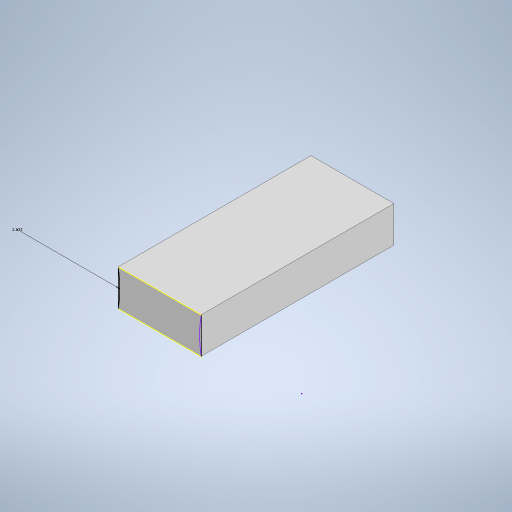
# Autodesk Inventor part: T610
Saved by Autodesk Inventor 2023 (Build 270158000, 158)
## iProperties
Created: 2023-01-25
Part Number: T610
Material: Generic
Document SubType Name: Modeling
Designer: abhim
Density: 1 g/cm^3
Appearance: Default
Author: abhim
Autodesk Inventor part; units mm, degrees
ref_plane "YZ Plane" through (0, 0, 0) normal (1, 0, 0) x (0, 1, 0)
ref_plane "XZ Plane" through (0, 0, 0) normal (0, 1, 0) x (-1, 0, 0)
ref_plane "XY Plane" through (0, 0, 0) normal (0, 0, 1) x (1, 0, 0)
sketch "Sketch1" plane through (0, 0, 0) normal (0, 1, 0) x (-1, 0, 0)
  line L0 (0, 0) -> (-43.942, 0)
  line L1 (-43.942, 0) -> (-43.942, -102.108)
  line L2 (-43.942, -102.108) -> (0, -102.108)
  line L3 (0, -102.108) -> (0, 0)
  dimension "d0" = 43.942
  dimension "d1" = 102.108
  constraints: 8 end point, 2 parallel, 1 horizontal, 1 perpendicular
  measures "d0" distance of L2.end L1.end
  measures "d1" distance of L1.end L0.end
extrude "Extrusion1" add sketch "Sketch1" along normal blind 19.05
sketch "Sketch2" plane through (0, 0, 0) normal (0, 0, 1) x (1, 0, 0)
  arc A0 (43.942, 19.05) -> (43.942, 0) centre (97.2787, 9.525) ccw
  line L0 (43.942, 0) -> (0, 0) projected
  line L1 (43.942, 19.05) -> (0, 19.05) projected
  arc A1 (0, 0) -> (0, 19.05) centre (-53.3343, 9.525) ccw
  line L2 (0, 19.05) -> (0, 0)
  line L3 (43.942, 19.05) -> (43.942, 0)
  dimension "d4" = 54.1782
  constraints: 4 end point, 4 point on circle, 2 centre point, 1 vertical
  measures "d4" radius of A1
body "Solid1"
